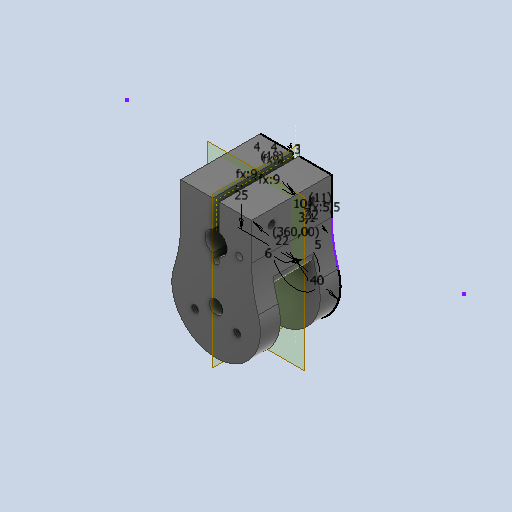
# Autodesk Inventor part: ParallelMech_DrivenPart_Motor_GC_ShaftConnector
Saved by Autodesk Inventor 2024 (Build 280153000, 153)
## iProperties
Created: 2022-08-03
Part Number: ParallelMech_DrivenPart_Motor_GC_ShaftConnector
Material: PBT-Kunststoff
Document SubType Name: Modeling
Designer: alexw
Density: 1.31 g/cm^3
Appearance: Glatt - Weiß
Mass: 62.503 g
Surface Area: 152.223 cm^2
Volume: 47.7122 cm^3
MotrGC_Part_OuterDia: 40,000 mm
FixationHole_Dia: 22,000 mm
SmallCapston_Offset: 25,000 mm
MotorFixation_Thickness: 18,000 mm
Author: alexw
Autodesk Inventor part; units mm, degrees
ref_plane "YZ Plane" through (0, 0, 0) normal (1, 0, 0) x (0, 1, 0)
ref_plane "XZ Plane" through (0, 0, 0) normal (0, 1, 0) x (-1, 0, 0)
ref_plane "XY Plane" through (0, 0, 0) normal (0, 0, 1) x (1, 0, 0)
sketch "Skizze1" plane through (0, 0, 0) normal (0, 0, 1) x (1, 0, 0)
  arc A0 (-1.5, 4.7697) -> (1.5, 4.7697) centre (0, 0) ccw
  arc A1 (-16, 0) -> (16, 0) centre (0, 0) ccw construction
  line L0 (-16, 0) -> (-16, 16.7697)
  line L1 (16, 16.7697) -> (16, 0)
  line L2 (-1.5, 16.7697) -> (-1.5, 4.7697)
  line L3 (1.5, 16.7697) -> (1.5, 4.7697)
  line L4 (-16, 16.7697) -> (-1.5, 16.7697)
  line L5 (1.5, 16.7697) -> (16, 16.7697)
  line L6 (-1.5, 4.7697) -> (1.5, 4.7697) construction
  line L7 (-16, 10.7697) -> (16, 10.7697) construction
  line L8 (-16, 8.7697) -> (16, 8.7697) construction
  line L9 (-16, 12.7697) -> (16, 12.7697) construction
  line L10 (-16, 0) -> (16, 0) construction
  line L11 (16, 0) -> (16, 0)
  line L12 (-16, 0) -> (-16, 0)
  line L13 (-16, 0) -> (16, 0) construction
  line L14 (16, 0) -> (-16, 0) construction
  circle A2 centre (0, -25) radius 20
  line L15 (0, 29.1236) -> (0, -57.3539) construction
  arc A3 (-19.0016, -18.7598) -> (-16, 0) centre (-76.125, 0) ccw
  arc A4 (16, 0) -> (19.0016, -18.7598) centre (76.125, 0) ccw
  circle A5 centre (0, -25) radius 11 construction
  circle A6 centre (0, -14) radius 2.5 construction
  circle A7 centre (0, -25) radius 3
  line L16 (1.5, 0) -> (-1.5, 0)
  line L17 (-1.5, 0) -> (-1.5, -7)
  arc A8 (-1.5, -7) -> (1.5, -7) centre (0, -7) ccw
  line L18 (1.5, -7) -> (1.5, 0)
  circle A9 centre (10.5, 0) radius 1.55
  point P0 (-1.5, 10.7697)
  point P1 (-9.5263, -30.5)
  point P2 (9.5263, -30.5)
  point P3 (12.5, 0)
  point P4 (-12.5, 0)
  point P5 (16, 0)
  point P6 (-16, 0)
  point P7 (0, -5)
  point P8 (0, 0)
  point P9 (1.5, -4.7697)
  point P10 (-1.5, -4.7697)
  point P11 (5, 0)
  dimension "FixationHole_Dia" = 22
  dimension "d0" = 10
  dimension "d1" = 32
  dimension "d2" = 3
  dimension "d3" = 4
  dimension "d4" = 2
  dimension "d5" = 4
  dimension "MotrGC_Part_OuterDia" = 40
  dimension "d8" = 5
  dimension "d12" = 360
  dimension "SmallCapston_Offset" = 25
  dimension "d51" = 6
  dimension "d53" = 7
  dimension "d68" = 11
  dimension "d69" = 5.5
  dimension "d70" = 3.1
  constraints: 36 end point, 13 point on circle, 12 perpendicular, 11 point on line, 9 centre point, 9 tangent, 6 coincident, 5 midpoint, 4 parallel, 2 collinear, 2 horizontal, 1 vertical, 1 vertical alignment, 6 other
  measures "d0" diameter of A0
  measures "d1" diameter of A1
  measures "d2" distance between parallel lines of L3 L2
  measures "d3" distance between parallel lines of L9 L8
  measures "d4" distance between parallel lines of L8 L7
  measures "d5" distance between parallel lines of L4 L9
  measures "MotrGC_Part_OuterDia" diameter of A2
  measures "d8" diameter of A6
  measures "SmallCapston_Offset" distance of point (0, 0) A2.centre
  measures "d51" diameter of A7
  measures "d53" distance of A0.centre A8.centre
  measures "d68" distance from line of L1 point (5, 0)
  measures "d69" distance from line of L1 point (10.5, 0)
  measures "d70" diameter of A9
extrude "Extrusion1" add sketch "Skizze1" along normal blind 36 contours A0 L17 A2 A3 L0 L4 L2 | L17 A8 L18 A2 | A0 L3 L5 L1 A4 A2 L18 | A9 picked at (-4.3164, -12.8926)
ref_plane "Arbeitsebene1" through (0, 0, 18) normal (0, 0, -1) x (-1, 0, 0)
sketch "Skizze4" plane through (0, 0, 18) normal (0, 0, -1) x (-1, 0, 0)
  arc A0 (-19.0016, -18.7598) -> (19.0016, -18.7598) centre (0, -25) ccw projected
  arc A1 (-19.0016, -18.7598) -> (19.0016, -18.7598) centre (0, -25) ccw projected
  arc A2 (-19.0016, -18.7598) -> (-16, 0) centre (-76.125, 0) ccw projected
  arc A3 (16, 0) -> (19.0016, -18.7598) centre (76.125, 0) ccw projected
  line L0 (-17.6527, -14) -> (17.6527, -14)
  point P0 (0, 0)
  dimension "d77" = 11
  constraints: 2 end point, 2 point on circle, 1 horizontal
  measures "d77" distance from line of L0 A0.centre
extrude "Extrusion2" cut sketch "Skizze4" along normal mid plane 18
hole "Bohrung1" at (-9.5263, -30.5, 0) at (9.5263, -30.5, 0) direction (0, 0, 1) diameter 4.5 depth 9 counterbore diameter 8 counterbore depth 4.5 clearance for "Inbusschraube DIN EN ISO 4762" size "M4" standard "DIN"
sketch "Skizze5" plane through (0, 0, 27) normal (0, 0, -1) x (-1, 0, 0)
  point P0 (0, 0)
  point P1 (-9.5263, -30.5)
  point P2 (9.5263, -30.5)
hole "Bohrung4" at (9.5263, -30.5, 27) at (-9.5263, -30.5, 27) direction (0, 0, 1) diameter 3.242 end through all thread size "M4x0.7" class "6H" standard "ISO Metric profile"
ref_plane "Arbeitsebene2" through (0, 0, 0) normal (-1, 0, 0) x (0, 0, 1)
sketch "Skizze2" plane through (0, 0, 0) normal (-1, 0, 0) x (0, 0, 1)
  line L0 (0, 16.7697) -> (0, 4.7697) construction
  line L1 (0, 4.7697) -> (36, 4.7697) construction
  line L2 (36, 16.7697) -> (36, 4.7697) construction
  line L3 (0, 16.7697) -> (36, 16.7697) construction
  line L4 (0, 10.7697) -> (36, 10.7697) construction
  line L5 (18, 10.7697) -> (18, 16.7697) construction
  point P0 (0, 0)
  point P1 (0, 10.7697)
  point P2 (0, 10.7697)
  point P3 (0, 10.7697)
  point P4 (9, 10.7697)
  point P5 (27, 10.7697)
  dimension "d24" = 18
  dimension "d25" = 9
  dimension "d26" = 9
  constraints: 4 end point, 4 midpoint, 2 point on line, 1 horizontal, 1 vertical
  measures "d24" distance between parallel lines of L5 L0
  measures "d25" distance from line of L5 point (9, 10.77)
  measures "d26" distance from line of L5 point (27, 10.77)
hole "Bohrung2" at (0, 10.7697, 27) at (0, 10.7697, 9) direction (1, 0, 0) diameter 3.242 end through all thread size "M4x0.7" class "6H" standard "ISO Metric profile"
sketch "Skizze3" plane through (-16, 0, 0) normal (-1, 0, 0) x (0, 0, 1)
  point P0 (0, 0)
  point P1 (9, 10.7697)
  point P2 (27, 10.7697)
hole "Bohrung3" at (-16, 10.7697, 9) at (-16, 10.7697, 27) direction (1, 0, 0) diameter 4.5 depth 14.5 counterbore diameter 8 counterbore depth 4.5 clearance for "Inbusschraube DIN EN ISO 4762" size "M4" standard "DIN"
fillet "Rundung1" radius 4 2 edges at (17.6527, -14, 18) (-17.6527, -14, 18)
extrude "Extrusion4" cut sketch "Skizze1" along normal through all contours A9
sketch "Skizze9" plane through (0, 0, 9) normal (0, 0, 1) x (1, 0, 0)
  circle A0 centre (9.5263, -30.5) radius 2.25 projected
  circle A1 centre (0, -25) radius 3 projected
  circle A2 centre (-9.5263, -30.5) radius 2.25 projected
  point P0 (0, 0)
extrude "Extrusion6" add sketch "Skizze9" against normal blind 0.5
sketch "Skizze6" plane through (16, 0, 0) normal (1, 0, 0) x (0, 0, -1)
  circle A0 centre (-27, 10.7697) radius 1.621 construction
  circle A1 centre (-9, 10.7697) radius 1.621 construction
  line L0 (0, 0) -> (0, 16.7697) construction
  line L1 (0, 16.7697) -> (-36, 16.7697) construction
  line L2 (-36, 0) -> (-36, 16.7697) construction
  line L3 (0, 0) -> (-36, 0) construction
  line L4 (-49, 16.7697) -> (13, 16.7697)
  line L5 (13, 16.7697) -> (13, 0)
  line L6 (13, 0) -> (-49, 0)
  line L7 (-49, 0) -> (-49, 16.7697)
  point P0 (0, 0)
  point P1 (-18, 16.7697)
  point P2 (-18, 0)
  dimension "d54" = 62
  constraints: 8 end point, 4 midpoint, 2 parallel, 1 horizontal, 1 perpendicular
  measures "d54" distance between parallel lines of L5 L7
sketch "Skizze7" plane through (26, 0, 0) normal (1, 0, 0) x (0, 0, -1)
  line L0 (-49, 50) -> (-49, -17) construction
  line L1 (-36, 50) -> (-36, -17) construction
  line L2 (0, 50) -> (0, -17) construction
  line L3 (13, 50) -> (13, -17) construction
  line L4 (-49, 16.7697) -> (-49, 0) construction
  line L5 (-49, 8.3848) -> (13, 8.3848) construction
  line L6 (13, 0) -> (13, 16.7697) projected
  point P0 (0, 0)
  point P1 (-42.5, 8.3848)
  point P2 (6.5, 8.3848)
  dimension "d58" = 13
  dimension "d59" = 6.5
  dimension "d60" = 6.5
  constraints: 2 end point, 2 midpoint, 2 point on line
  measures "d58" distance between parallel lines of L1 L0
  measures "d59" distance from line of L0 point (-42.5, 8.385)
  measures "d60" distance from line of L3 point (6.5, 8.385)
equation "\"d4\" = 0.5 * d3"
equation "\"d69\" = 0.5 * d68"
equation "\"d25\" = 0.5 * d24"
equation "\"d26\" = 0.5 * d24"
equation "\"d59\" = 0.5 * d58"
equation "\"d60\" = d59"
